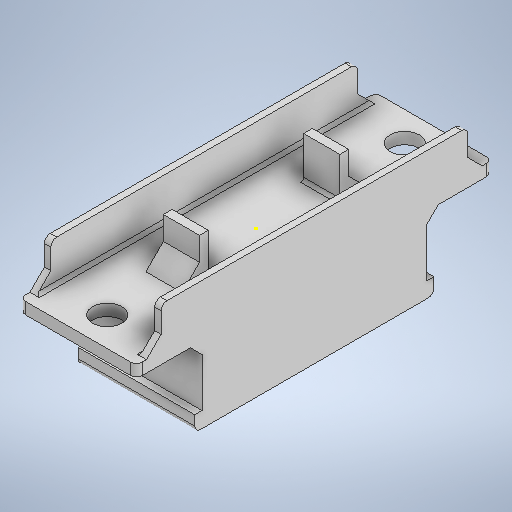
# Autodesk Inventor part: Platte 3V3 modul
Saved by Autodesk Inventor 2025.2 (Build 292293000, 293)
## iProperties
Created: 2025-03-23
Part Number: Platte 3V3 modul
Material: Generisch
Document SubType Name: Modeling
Designer: Quatana
Density: 1 g/cm^3
Appearance: Vorgabe
Author: Quatana
## iProperties of the stored document Relais_Platte_3D-Druck.ipt
Created: 2025-03-23
Part Number: Relais_Platte_3D-Druck
Material: Generisch
Document SubType Name: Modeling
Designer: Quatana
Density: 1 g/cm^3
Appearance: Vorgabe
Author: Quatana
Autodesk Inventor part; units mm, degrees
ref_plane "YZ Plane" through (0, 0, 0) normal (1, 0, 0) x (0, 1, 0)
ref_plane "XZ Plane" through (0, 0, 0) normal (0, 1, 0) x (-1, 0, 0)
ref_plane "XY Plane" through (0, 0, 0) normal (0, 0, 1) x (1, 0, 0)
sketch "Skizze1" plane through (0, 0, 0) normal (0, 0, 1) x (1, 0, 0)
  line L0 (-10, -30.5) -> (10, -30.5)
  line L1 (10, -30.5) -> (10, 30.5)
  line L2 (10, 30.5) -> (-10, 30.5)
  line L3 (-10, 30.5) -> (-10, -30.5)
  line L4 (-10, -30.5) -> (10, 30.5) construction
  line L5 (10, -30.5) -> (-10, 30.5) construction
  point P0 (0, 0)
  dimension "d0" = 20
  dimension "d1" = 61
  constraints: 12 end point, 2 midpoint, 2 parallel, 1 horizontal, 1 perpendicular
  measures "d0" distance of L2.end L1.end
  measures "d1" distance of L1.end L0.end
extrude "Extrusion1" add sketch "Skizze1" along normal blind 2
sketch "Skizze3" plane through (0, 0, 0) normal (0, 0, -1) x (-1, 0, 0)
  line L0 (10, 30.5) -> (10, -30.5) projected
  line L1 (-10, -20.5) -> (10, -20.5)
  line L2 (10, -20.5) -> (10, 20.5)
  line L3 (10, 20.5) -> (-10, 20.5)
  line L4 (-10, 20.5) -> (-10, -20.5)
  line L5 (-10, -20.5) -> (10, 20.5) construction
  line L6 (10, -20.5) -> (-10, 20.5) construction
  line L7 (10, -30.5) -> (-10, -30.5) projected
  line L8 (-10, -30.5) -> (-10, 30.5) projected
  point P0 (0, 0)
  point P1 (10, -20.5)
  dimension "d9" = 41
  dimension "d17" = 10
  constraints: 12 end point, 2 midpoint, 2 parallel, 1 horizontal, 1 perpendicular, 1 point on line, 1 vertical alignment
  measures "d9" distance between parallel lines of L1 L3
  measures "d17" distance between parallel lines of L7 L1
extrude "Extrusion3" add sketch "Skizze3" along normal blind 13 contours L0 L1 L4 L3
sketch "Skizze4" plane through (-10, -30.5, 2) normal (-1, 0, 0) x (0, 0, 1)
  line L0 (-2, 10) -> (-15, 10) projected
  line L1 (-12.32, 10) -> (-2, 10)
  line L2 (-2, 10) -> (-2, 11.25)
  line L3 (-2, 11.25) -> (-12.32, 11.25)
  line L4 (-12.32, 11.25) -> (-12.32, 10)
  line L5 (-15, 10) -> (-15, 51) projected
  line L6 (-4.404, 30.5) -> (2.981, 30.5) construction
  line L7 (-2, 51) -> (-15, 51)
  line L8 (-2, 51) -> (-2, 49.75)
  line L9 (-2, 49.75) -> (-12.32, 49.75)
  line L10 (-12.32, 49.75) -> (-12.32, 51)
  line L11 (-2, 10) -> (-12.32, 10)
  point P0 (-2, 30.5)
  point P1 (-12.32, 10.625)
  dimension "d12" = 2.68
  dimension "d13" = 1.25
  constraints: 20 end point, 5 symmetric about line, 3 point on line, 2 horizontal, 2 parallel, 1 collinear, 1 midpoint, 1 perpendicular
  measures "d12" distance from line of L5 point (-12.32, 10.625)
  measures "d13" distance between parallel lines of L3 L0
extrude "Extrusion4" cut sketch "Skizze4" against normal through all
fillet "Rundung1" radius 1 6 edges at (-10, -30.5, 1) (10, -30.5, 1) (10, 30.5, 1) (-10, 30.5, 1) (0, 20.5, -13) (0, -20.5, -13)
sketch "Skizze6" plane through (0, 0, 2) normal (0, 0, 1) x (1, 0, 0)
  point P0 (0, 0)
sketch "Skizze7" plane through (0, 0, 2) normal (0, 0, 1) x (1, 0, 0)
  line L0 (-8.9, 11.275) -> (8.9, 11.275)
  line L1 (8.9, 11.275) -> (8.9, -11.275)
  line L2 (8.9, -11.275) -> (-8.9, -11.275)
  line L3 (-8.9, -11.275) -> (-8.9, 11.275)
  line L4 (-8.9, 11.275) -> (8.9, -11.275) construction
  line L5 (8.9, 11.275) -> (-8.9, -11.275) construction
  line L6 (-8.9, 11.275) -> (-10, 11.275)
  line L7 (-10, 11.275) -> (-10, -11.275)
  line L8 (-10, -11.275) -> (-8.9, -11.275)
  line L9 (8.9, 11.275) -> (10, 11.275)
  line L10 (10, 11.275) -> (10, -11.275)
  line L11 (10, -11.275) -> (8.9, -11.275)
  line L12 (10, -29.5) -> (10, 29.5) projected
  line L13 (-10, 29.5) -> (-10, -29.5) projected
  line L14 (-3.1, 12.775) -> (3.1, 12.775)
  line L15 (3.1, 12.775) -> (3.1, 11.275)
  line L16 (3.1, 11.275) -> (-3.1, 11.275)
  line L17 (-3.1, 11.275) -> (-3.1, 12.775)
  line L18 (-3.1, 12.775) -> (3.1, 11.275) construction
  line L19 (3.1, 12.775) -> (-3.1, 11.275) construction
  line L20 (-0.8378, 0) -> (1.8317, 0) construction
  line L21 (-3.1, -12.775) -> (3.1, -12.775)
  line L22 (3.1, -12.775) -> (3.1, -11.275)
  line L23 (3.1, -11.275) -> (-3.1, -11.275)
  line L24 (-3.1, -11.275) -> (-3.1, -12.775)
  line L25 (10, 11.275) -> (8.9, 11.275)
  line L26 (8.9, 11.275) -> (8.9, 26.275)
  line L27 (8.9, 26.275) -> (10, 26.275)
  line L28 (10, 26.275) -> (10, 11.275)
  line L29 (0, 1.7909) -> (0, -1.8992) construction
  line L30 (8.9, -11.275) -> (10, -11.275)
  line L31 (10, 29.5) -> (10, -29.5)
  line L32 (8.9, -11.275) -> (8.9, -26.275)
  line L33 (8.9, -26.275) -> (10, -26.275)
  line L34 (-8.9, 11.275) -> (-10, 11.275)
  line L35 (-10, -11.275) -> (-8.9, -11.275)
  line L36 (-10, -29.5) -> (-10, 29.5)
  line L37 (-8.9, 11.275) -> (-8.9, 26.275)
  line L38 (-8.9, 26.275) -> (-10, 26.275)
  line L39 (-8.9, -11.275) -> (-8.9, -26.275)
  line L40 (-8.9, -26.275) -> (-10, -26.275)
  point P0 (0, 0)
  point P1 (0, 0)
  point P2 (0, 12.025)
  point P3 (8.9, 18.775)
  dimension "d36" = 17.8
  dimension "d37" = 22.55
  dimension "d38" = 6.2
  dimension "d39" = 1.5
  dimension "d45" = 15
  constraints: 78 end point, 17 symmetric about line, 8 point on line, 7 parallel, 5 midpoint, 5 perpendicular, 4 horizontal, 2 vertical alignment, 1 coincident, 1 collinear
  measures "d36" distance of L1.end L2.end
  measures "d37" distance of L0.end L1.end
  measures "d38" distance of L15.end L16.end
  measures "d39" distance of L14.end L15.end
  measures "d45" distance of L0.end L26.end
extrude "Extrusion5" add sketch "Skizze7" along normal blind 7 contours L3 L8 L7 L6 | L6 L13 L38 L37 | L17 L14 L15 L0 | L39 L40 L13 L8 | L2 L22 L21 L24 | L9 L10 L11 L1 | L26 L27 L12 L9 | L11 L12 L33 L32
chamfer "Fasen1" distance 2 angle 45 2 edges at (0, -19.25, 0) (0, 19.25, 0)
chamfer "Fasen2" distance 3 angle 45 2 edges at (0, 12.775, 2) (0, -12.775, 2)
chamfer "Fasen3" distance 2.5 angle 45 4 edges at (9.45, -26.275, 2) (-9.45, -26.275, 2) (-9.45, 26.275, 2) (9.45, 26.275, 2)
sketch "Skizze8" plane through (0, 0, 2) normal (0, 0, 1) x (1, 0, 0)
  circle A0 centre (0, 25.5) radius 2.5
  line L0 (1.3354, 0) -> (-2.5, 0) construction
  circle A1 centre (0, -25.5) radius 2.5
  line L1 (9, 30.5) -> (-9, 30.5) projected
  point P0 (0, 0)
  point P1 (0, 30.5)
  dimension "d52" = 5
  dimension "d55" = 5
  constraints: 2 centre point, 2 end point, 1 horizontal, 1 midpoint, 1 symmetric about line, 1 vertical alignment, 1 other
  measures "d52" diameter of A0
  measures "d55" distance of point (0, 30.5) A0.centre
extrude "Extrusion6" cut sketch "Skizze8" against normal through all
fillet "Rundung2" radius 1 4 edges at (-9.45, -26.275, 9) (9.45, -26.275, 9) (-9.45, 26.275, 9) (9.45, 26.275, 9)
fillet "Rundung3" radius 0.5 2 edges at (-8.9, 0, 2) (8.9, 0, 2)
fillet "Rundung4" radius 0.5 2 edges at (0, -11.275, 2) (0, 11.275, 2)
